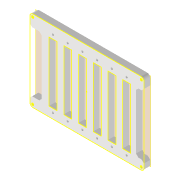
# Autodesk Inventor part: Omniscope_USBC_Base_Top+
Saved by Autodesk Inventor 2022 (Build 260153000, 153)
## iProperties
Created: 2023-05-17
Part Number: Omniscope_USBC_Base_Top+
Material: Generisch
Document SubType Name: Modeling
Designer: diederichbenedict
Density: 1 g/cm^3
Appearance: Vorgabe
Author: diederichbenedict
Autodesk Inventor part; units mm, degrees
(part 1 of 3)
ref_plane "YZ Plane" through (0, 0, 0) normal (1, 0, 0) x (0, 1, 0)
ref_plane "XZ Plane" through (0, 0, 0) normal (0, 1, 0) x (-1, 0, 0)
ref_plane "XY Plane" through (0, 0, 0) normal (0, 0, 1) x (1, 0, 0)
ref_plane "Arbeitsebene1" through (0, 0, 0) normal (0, 0, 1) x (1, 0, 0)
sketch "Skizze1" plane through (0, 0, 0) normal (0, 0, 1) x (1, 0, 0)
  line L0 (12.3616, -8.1796) -> (13.1516, -8.1796) projected
  line L1 (13.1516, -8.1796) -> (13.1516, -8.5796) projected
  line L2 (13.1516, -8.5796) -> (12.3616, -8.5796) projected
  line L3 (12.3616, -8.5796) -> (12.3616, -8.1796) projected
  line L4 (12.3616, -8.9796) -> (13.1516, -8.9796) projected
  line L5 (13.1516, -8.9796) -> (13.1516, -9.3796) projected
  line L6 (13.1516, -9.3796) -> (12.3616, -9.3796) projected
  line L7 (12.3616, -9.3796) -> (12.3616, -8.9796) projected
  line L8 (9.9166, -12.9796) -> (9.9166, -12.5796) projected
  line L9 (9.9166, -12.5796) -> (9.8216, -12.5796) projected
  line L10 (9.8216, -12.5796) -> (9.8216, -12.1796) projected
  line L11 (9.8216, -12.1796) -> (9.9166, -12.1796) projected
  line L12 (9.9166, -12.1796) -> (9.9166, -11.7796) projected
  line L13 (9.9166, -11.7796) -> (9.8216, -11.7796) projected
  line L14 (9.8216, -11.7796) -> (9.8216, -11.3796) projected
  line L15 (9.8216, -11.3796) -> (9.9166, -11.3796) projected
  line L16 (9.9166, -11.3796) -> (9.9166, -10.9796) projected
  line L17 (9.9166, -10.9796) -> (9.8216, -10.9796) projected
  line L18 (9.8216, -10.9796) -> (9.8216, -10.5796) projected
  line L19 (9.8216, -10.5796) -> (9.9166, -10.5796) projected
  line L20 (9.9166, -10.5796) -> (9.9166, -10.1796) projected
  line L21 (9.9166, -10.1796) -> (9.8216, -10.1796) projected
  line L22 (9.8216, -10.1796) -> (9.8216, -9.7796) projected
  line L23 (9.8216, -9.7796) -> (9.9166, -9.7796) projected
  line L24 (9.9166, -9.7796) -> (9.9166, -9.3796) projected
  line L25 (9.9166, -9.3796) -> (9.8216, -9.3796) projected
  line L26 (9.8216, -9.3796) -> (9.8216, -8.9796) projected
  line L27 (9.8216, -8.9796) -> (9.9166, -8.9796) projected
  line L28 (9.9166, -8.9796) -> (9.9166, -8.5796) projected
  line L29 (9.9166, -8.5796) -> (9.8216, -8.5796) projected
  line L30 (9.8216, -8.5796) -> (9.8216, -8.1796) projected
  line L31 (9.8216, -8.1796) -> (9.9166, -8.1796) projected
  line L32 (9.9166, -8.1796) -> (9.9166, -8.0296) projected
  arc A0 (10.6866, -6.9803) -> (9.9166, -8.0296) centre (11.0166, -8.0296) ccw projected
  line L33 (10.6866, -6.9803) -> (10.6866, -6.9046) projected
  line L34 (10.6866, -6.9046) -> (12.2866, -6.9046) projected
  line L35 (12.2866, -6.9046) -> (12.2866, -7.5546) projected
  line L36 (12.2866, -7.5546) -> (12.0088, -7.5546) projected
  arc A1 (12.1166, -8.0296) -> (12.0088, -7.5546) centre (11.0166, -8.0296) ccw projected
  line L37 (12.1166, -8.0296) -> (12.1166, -13.9296) projected
  arc A2 (11.6832, -14.8046) -> (12.1166, -13.9296) centre (11.0166, -13.9296) ccw projected
  line L38 (11.6832, -14.8046) -> (12.2866, -14.8046) projected
  line L39 (12.2866, -14.8046) -> (12.2866, -15.4546) projected
  line L40 (12.2866, -15.4546) -> (10.6866, -15.4546) projected
  line L41 (10.6866, -15.4546) -> (10.6866, -14.9789) projected
  arc A3 (9.9454, -14.1796) -> (10.6866, -14.9789) centre (11.0166, -13.9296) ccw projected
  line L42 (9.9454, -14.1796) -> (9.8216, -14.1796) projected
  line L43 (9.8216, -14.1796) -> (9.8216, -13.7796) projected
  line L44 (9.8216, -13.7796) -> (9.9166, -13.7796) projected
  line L45 (9.9166, -13.7796) -> (9.9166, -13.3796) projected
  line L46 (9.9166, -13.3796) -> (9.8216, -13.3796) projected
  line L47 (9.8216, -13.3796) -> (9.8216, -12.9796) projected
  line L48 (9.8216, -12.9796) -> (9.9166, -12.9796) projected
  line L49 (12.3616, -9.7796) -> (13.1516, -9.7796) projected
  line L50 (13.1516, -9.7796) -> (13.1516, -10.1796) projected
  line L51 (13.1516, -10.1796) -> (12.3616, -10.1796) projected
  line L52 (12.3616, -10.1796) -> (12.3616, -9.7796) projected
  line L53 (12.3616, -10.5796) -> (13.1516, -10.5796) projected
  line L54 (13.1516, -10.5796) -> (13.1516, -10.9796) projected
  line L55 (13.1516, -10.9796) -> (12.3616, -10.9796) projected
  line L56 (12.3616, -10.9796) -> (12.3616, -10.5796) projected
  line L57 (12.3616, -11.3796) -> (13.1516, -11.3796) projected
  line L58 (13.1516, -11.3796) -> (13.1516, -11.7796) projected
  line L59 (13.1516, -11.7796) -> (12.3616, -11.7796) projected
  line L60 (12.3616, -11.7796) -> (12.3616, -11.3796) projected
  line L61 (12.3616, -12.1796) -> (13.1516, -12.1796) projected
  line L62 (13.1516, -12.1796) -> (13.1516, -12.5796) projected
  line L63 (13.1516, -12.5796) -> (12.3616, -12.5796) projected
  line L64 (12.3616, -12.5796) -> (12.3616, -12.1796) projected
  line L65 (12.3616, -12.9796) -> (13.1516, -12.9796) projected
  line L66 (13.1516, -12.9796) -> (13.1516, -13.3796) projected
  line L67 (13.1516, -13.3796) -> (12.3616, -13.3796) projected
  line L68 (12.3616, -13.3796) -> (12.3616, -12.9796) projected
  line L69 (12.3616, -13.7796) -> (13.1516, -13.7796) projected
  line L70 (13.1516, -13.7796) -> (13.1516, -14.1796) projected
  line L71 (13.1516, -14.1796) -> (12.3616, -14.1796) projected
  line L72 (12.3616, -14.1796) -> (12.3616, -13.7796) projected
  line L73 (-47.0034, 29.7204) -> (-46.2134, 29.7204) projected
  line L74 (-46.2134, 29.7204) -> (-46.2134, 29.3204) projected
  line L75 (-46.2134, 29.3204) -> (-47.0034, 29.3204) projected
  line L76 (-47.0034, 29.3204) -> (-47.0034, 29.7204) projected
  line L77 (-47.0034, 28.9204) -> (-46.2134, 28.9204) projected
  line L78 (-46.2134, 28.9204) -> (-46.2134, 28.5204) projected
  line L79 (-46.2134, 28.5204) -> (-47.0034, 28.5204) projected
  line L80 (-47.0034, 28.5204) -> (-47.0034, 28.9204) projected
  line L81 (-47.0034, 28.1204) -> (-46.2134, 28.1204) projected
  line L82 (-46.2134, 28.1204) -> (-46.2134, 27.7204) projected
  line L83 (-46.2134, 27.7204) -> (-47.0034, 27.7204) projected
  line L84 (-47.0034, 27.7204) -> (-47.0034, 28.1204) projected
  line L85 (-47.0034, 27.3204) -> (-46.2134, 27.3204) projected
  line L86 (-46.2134, 27.3204) -> (-46.2134, 26.9204) projected
  line L87 (-46.2134, 26.9204) -> (-47.0034, 26.9204) projected
  line L88 (-47.0034, 26.9204) -> (-47.0034, 27.3204) projected
  line L89 (-47.0034, 26.5204) -> (-46.2134, 26.5204) projected
  line L90 (-46.2134, 26.5204) -> (-46.2134, 26.1204) projected
  line L91 (-46.2134, 26.1204) -> (-47.0034, 26.1204) projected
  line L92 (-47.0034, 26.1204) -> (-47.0034, 26.5204) projected
  line L93 (-47.0034, 25.7204) -> (-46.2134, 25.7204) projected
  line L94 (-46.2134, 25.7204) -> (-46.2134, 25.3204) projected
  line L95 (-46.2134, 25.3204) -> (-47.0034, 25.3204) projected
  line L96 (-47.0034, 25.3204) -> (-47.0034, 25.7204) projected
  line L97 (-47.0034, 24.9204) -> (-46.2134, 24.9204) projected
  line L98 (-46.2134, 24.9204) -> (-46.2134, 24.5204) projected
  line L99 (-46.2134, 24.5204) -> (-47.0034, 24.5204) projected
  line L100 (-47.0034, 24.5204) -> (-47.0034, 24.9204) projected
  line L101 (-47.0034, 24.1204) -> (-46.2134, 24.1204) projected
  line L102 (-46.2134, 24.1204) -> (-46.2134, 23.7204) projected
  line L103 (-46.2134, 23.7204) -> (-47.0034, 23.7204) projected
  line L104 (-47.0034, 23.7204) -> (-47.0034, 24.1204) projected
  line L105 (49.9241, -8.1296) -> (50.7141, -8.1296) projected
  line L106 (50.7141, -8.1296) -> (50.7141, -8.5296) projected
  line L107 (50.7141, -8.5296) -> (49.9241, -8.5296) projected
  line L108 (49.9241, -8.5296) -> (49.9241, -8.1296) projected
  line L109 (49.9241, -8.9296) -> (50.7141, -8.9296) projected
  line L110 (50.7141, -8.9296) -> (50.7141, -9.3296) projected
  line L111 (50.7141, -9.3296) -> (49.9241, -9.3296) projected
  line L112 (49.9241, -9.3296) -> (49.9241, -8.9296) projected
  line L113 (49.9241, -9.7296) -> (50.7141, -9.7296) projected
  line L114 (50.7141, -9.7296) -> (50.7141, -10.1296) projected
  line L115 (50.7141, -10.1296) -> (49.9241, -10.1296) projected
  line L116 (49.9241, -10.1296) -> (49.9241, -9.7296) projected
  line L117 (49.9241, -10.5296) -> (50.7141, -10.5296) projected
  line L118 (50.7141, -10.5296) -> (50.7141, -10.9296) projected
  line L119 (50.7141, -10.9296) -> (49.9241, -10.9296) projected
  line L120 (49.9241, -10.9296) -> (49.9241, -10.5296) projected
  line L121 (49.9241, -11.3296) -> (50.7141, -11.3296) projected
  line L122 (50.7141, -11.3296) -> (50.7141, -11.7296) projected
  line L123 (50.7141, -11.7296) -> (49.9241, -11.7296) projected
  line L124 (49.9241, -11.7296) -> (49.9241, -11.3296) projected
  line L125 (49.9241, -12.1296) -> (50.7141, -12.1296) projected
  line L126 (50.7141, -12.1296) -> (50.7141, -12.5296) projected
  line L127 (50.7141, -12.5296) -> (49.9241, -12.5296) projected
  line L128 (49.9241, -12.5296) -> (49.9241, -12.1296) projected
  line L129 (49.9241, -12.9296) -> (50.7141, -12.9296) projected
  line L130 (50.7141, -12.9296) -> (50.7141, -13.3296) projected
  line L131 (50.7141, -13.3296) -> (49.9241, -13.3296) projected
  line L132 (49.9241, -13.3296) -> (49.9241, -12.9296) projected
  line L133 (49.9241, -13.7296) -> (50.7141, -13.7296) projected
  line L134 (50.7141, -13.7296) -> (50.7141, -14.1296) projected
  line L135 (50.7141, -14.1296) -> (49.9241, -14.1296) projected
  line L136 (49.9241, -14.1296) -> (49.9241, -13.7296) projected
  arc A4 (49.5166, -8.0296) -> (49.3832, -7.5046) centre (48.4166, -8.0296) ccw projected
  line L137 (49.5166, -8.0296) -> (49.5166, -13.9296) projected
  arc A5 (49.1442, -14.7546) -> (49.5166, -13.9296) centre (48.4166, -13.9296) ccw projected
  line L138 (49.1442, -14.7546) -> (49.8491, -14.7546) projected
  line L139 (49.8491, -14.7546) -> (49.8491, -15.4046) projected
  line L140 (49.8491, -15.4046) -> (48.2491, -15.4046) projected
  line L141 (48.2491, -15.4046) -> (48.2491, -15.0168) projected
  arc A6 (47.3166, -13.9296) -> (48.2491, -15.0168) centre (48.4166, -13.9296) ccw projected
  line L142 (47.3166, -13.9296) -> (47.3166, -8.0296) projected
  arc A7 (48.2491, -6.9424) -> (47.3166, -8.0296) centre (48.4166, -8.0296) ccw projected
  line L143 (48.2491, -6.9424) -> (48.2491, -6.8546) projected
  line L144 (48.2491, -6.8546) -> (49.8491, -6.8546) projected
  line L145 (49.8491, -6.8546) -> (49.8491, -7.5046) projected
  line L146 (49.8491, -7.5046) -> (49.3832, -7.5046) projected
  line L147 (-46.1834, -8.0546) -> (-46.1834, -8.0296) projected
  arc A8 (-46.0054, -7.4296) -> (-46.1834, -8.0296) centre (-45.0834, -8.0296) ccw projected
  line L148 (-46.0054, -7.4296) -> (-46.0634, -7.4296) projected
  line L149 (-46.0634, -7.4296) -> (-46.0634, -6.7796) projected
  line L150 (-46.0634, -6.7796) -> (-44.4634, -6.7796) projected
  line L151 (-44.4634, -6.7796) -> (-44.4634, -7.121) projected
  arc A9 (-43.9834, -8.0296) -> (-44.4634, -7.121) centre (-45.0834, -8.0296) ccw projected
  line L152 (-43.9834, -8.0296) -> (-43.9834, -8.0546) projected
  line L153 (-43.9834, -8.0546) -> (-43.5984, -8.0546) projected
  line L154 (-43.5984, -8.0546) -> (-43.5984, -8.4546) projected
  line L155 (-43.5984, -8.4546) -> (-43.9834, -8.4546) projected
  line L156 (-43.9834, -8.4546) -> (-43.9834, -8.8546) projected
  line L157 (-43.9834, -8.8546) -> (-43.5984, -8.8546) projected
  line L158 (-43.5984, -8.8546) -> (-43.5984, -9.2546) projected
  line L159 (-43.5984, -9.2546) -> (-43.9834, -9.2546) projected
  line L160 (-43.9834, -9.2546) -> (-43.9834, -9.6546) projected
  line L161 (-43.9834, -9.6546) -> (-43.5984, -9.6546) projected
  line L162 (-43.5984, -9.6546) -> (-43.5984, -10.0546) projected
  line L163 (-43.5984, -10.0546) -> (-43.9834, -10.0546) projected
  line L164 (-43.9834, -10.0546) -> (-43.9834, -10.4546) projected
  line L165 (-43.9834, -10.4546) -> (-43.5984, -10.4546) projected
  line L166 (-43.5984, -10.4546) -> (-43.5984, -10.8546) projected
  line L167 (-43.5984, -10.8546) -> (-43.9834, -10.8546) projected
  line L168 (-43.9834, -10.8546) -> (-43.9834, -11.2546) projected
  line L169 (-43.9834, -11.2546) -> (-43.5984, -11.2546) projected
  line L170 (-43.5984, -11.2546) -> (-43.5984, -11.6546) projected
  line L171 (-43.5984, -11.6546) -> (-43.9834, -11.6546) projected
  line L172 (-43.9834, -11.6546) -> (-43.9834, -12.0546) projected
  line L173 (-43.9834, -12.0546) -> (-43.5984, -12.0546) projected
  line L174 (-43.5984, -12.0546) -> (-43.5984, -12.4546) projected
  line L175 (-43.5984, -12.4546) -> (-43.9834, -12.4546) projected
  line L176 (-43.9834, -12.4546) -> (-43.9834, -12.8546) projected
  line L177 (-43.9834, -12.8546) -> (-43.5984, -12.8546) projected
  line L178 (-43.5984, -12.8546) -> (-43.5984, -13.2546) projected
  line L179 (-43.5984, -13.2546) -> (-43.9834, -13.2546) projected
  line L180 (-43.9834, -13.2546) -> (-43.9834, -13.6546) projected
  line L181 (-43.9834, -13.6546) -> (-43.5984, -13.6546) projected
  line L182 (-43.5984, -13.6546) -> (-43.5984, -14.0546) projected
  line L183 (-43.5984, -14.0546) -> (-43.9905, -14.0546) projected
  arc A10 (-44.4634, -14.8382) -> (-43.9905, -14.0546) centre (-45.0834, -13.9296) ccw projected
  line L184 (-44.4634, -14.8382) -> (-44.4634, -15.3296) projected
  line L185 (-44.4634, -15.3296) -> (-46.0634, -15.3296) projected
  line L186 (-46.0634, -15.3296) -> (-46.0634, -14.6796) projected
  line L187 (-46.0634, -14.6796) -> (-45.8881, -14.6796) projected
  arc A11 (-46.1763, -14.0546) -> (-45.8881, -14.6796) centre (-45.0834, -13.9296) ccw projected
  line L188 (-46.1763, -14.0546) -> (-46.9284, -14.0546) projected
  line L189 (-46.9284, -14.0546) -> (-46.9284, -13.6546) projected
  line L190 (-46.9284, -13.6546) -> (-46.1834, -13.6546) projected
  line L191 (-46.1834, -13.6546) -> (-46.1834, -13.2546) projected
  line L192 (-46.1834, -13.2546) -> (-46.9284, -13.2546) projected
  line L193 (-46.9284, -13.2546) -> (-46.9284, -12.8546) projected
  line L194 (-46.9284, -12.8546) -> (-46.1834, -12.8546) projected
  line L195 (-46.1834, -12.8546) -> (-46.1834, -12.4546) projected
  line L196 (-46.1834, -12.4546) -> (-46.9284, -12.4546) projected
  line L197 (-46.9284, -12.4546) -> (-46.9284, -12.0546) projected
  line L198 (-46.9284, -12.0546) -> (-46.1834, -12.0546) projected
  line L199 (-46.1834, -12.0546) -> (-46.1834, -11.6546) projected
  line L200 (-46.1834, -11.6546) -> (-46.9284, -11.6546) projected
  line L201 (-46.9284, -11.6546) -> (-46.9284, -11.2546) projected
  line L202 (-46.9284, -11.2546) -> (-46.1834, -11.2546) projected
  line L203 (-46.1834, -11.2546) -> (-46.1834, -10.8546) projected
  line L204 (-46.1834, -10.8546) -> (-46.9284, -10.8546) projected
  line L205 (-46.9284, -10.8546) -> (-46.9284, -10.4546) projected
  line L206 (-46.9284, -10.4546) -> (-46.1834, -10.4546) projected
  line L207 (-46.1834, -10.4546) -> (-46.1834, -10.0546) projected
  line L208 (-46.1834, -10.0546) -> (-46.9284, -10.0546) projected
  line L209 (-46.9284, -10.0546) -> (-46.9284, -9.6546) projected
  line L210 (-46.9284, -9.6546) -> (-46.1834, -9.6546) projected
  line L211 (-46.1834, -9.6546) -> (-46.1834, -9.2546) projected
  line L212 (-46.1834, -9.2546) -> (-46.9284, -9.2546) projected
  line L213 (-46.9284, -9.2546) -> (-46.9284, -8.8546) projected
  line L214 (-46.9284, -8.8546) -> (-46.1834, -8.8546) projected
  line L215 (-46.1834, -8.8546) -> (-46.1834, -8.4546) projected
  line L216 (-46.1834, -8.4546) -> (-46.9284, -8.4546) projected
  line L217 (-46.9284, -8.4546) -> (-46.9284, -8.0546) projected
  line L218 (-46.9284, -8.0546) -> (-46.1834, -8.0546) projected
  line L219 (31.8441, -32.7296) -> (31.0541, -32.7296) projected
  line L220 (31.0541, -32.7296) -> (31.0541, -32.3296) projected
  line L221 (31.0541, -32.3296) -> (31.8441, -32.3296) projected
  line L222 (31.8441, -32.3296) -> (31.8441, -32.7296) projected
  line L223 (31.8441, -31.9296) -> (31.0541, -31.9296) projected
  line L224 (31.0541, -31.9296) -> (31.0541, -31.5296) projected
  line L225 (31.0541, -31.5296) -> (31.8441, -31.5296) projected
  line L226 (31.8441, -31.5296) -> (31.8441, -31.9296) projected
  line L227 (31.8441, -31.1296) -> (31.0541, -31.1296) projected
  line L228 (31.0541, -31.1296) -> (31.0541, -30.7296) projected
  line L229 (31.0541, -30.7296) -> (31.8441, -30.7296) projected
  line L230 (31.8441, -30.7296) -> (31.8441, -31.1296) projected
  line L231 (31.8441, -30.3296) -> (31.0541, -30.3296) projected
  line L232 (31.0541, -30.3296) -> (31.0541, -29.9296) projected
  line L233 (31.0541, -29.9296) -> (31.8441, -29.9296) projected
  line L234 (31.8441, -29.9296) -> (31.8441, -30.3296) projected
  line L235 (31.8441, -29.5296) -> (31.0541, -29.5296) projected
  line L236 (31.0541, -29.5296) -> (31.0541, -29.1296) projected
  line L237 (31.0541, -29.1296) -> (31.8441, -29.1296) projected
  line L238 (31.8441, -29.1296) -> (31.8441, -29.5296) projected
  line L239 (31.8441, -28.7296) -> (31.0541, -28.7296) projected
  line L240 (31.0541, -28.7296) -> (31.0541, -28.3296) projected
  line L241 (31.0541, -28.3296) -> (31.8441, -28.3296) projected
  line L242 (31.8441, -28.3296) -> (31.8441, -28.7296) projected
  line L243 (31.8441, -27.9296) -> (31.0541, -27.9296) projected
  line L244 (31.0541, -27.9296) -> (31.0541, -27.5296) projected
  line L245 (31.0541, -27.5296) -> (31.8441, -27.5296) projected
  line L246 (31.8441, -27.5296) -> (31.8441, -27.9296) projected
  line L247 (31.8441, -27.1296) -> (31.0541, -27.1296) projected
  line L248 (31.0541, -27.1296) -> (31.0541, -26.7296) projected
  line L249 (31.0541, -26.7296) -> (31.8441, -26.7296) projected
  line L250 (31.8441, -26.7296) -> (31.8441, -27.1296) projected
  line L251 (50.8941, -32.7546) -> (50.1041, -32.7546) projected
  line L252 (50.1041, -32.7546) -> (50.1041, -32.3546) projected
  line L253 (50.1041, -32.3546) -> (50.8941, -32.3546) projected
  line L254 (50.8941, -32.3546) -> (50.8941, -32.7546) projected
  line L255 (50.8941, -31.9546) -> (50.1041, -31.9546) projected
  line L256 (50.1041, -31.9546) -> (50.1041, -31.5546) projected
  line L257 (50.1041, -31.5546) -> (50.8941, -31.5546) projected
  line L258 (50.8941, -31.5546) -> (50.8941, -31.9546) projected
  line L259 (50.8941, -31.1546) -> (50.1041, -31.1546) projected
  line L260 (50.1041, -31.1546) -> (50.1041, -30.7546) projected
  line L261 (50.1041, -30.7546) -> (50.8941, -30.7546) projected
  line L262 (50.8941, -30.7546) -> (50.8941, -31.1546) projected
  line L263 (50.8941, -30.3546) -> (50.1041, -30.3546) projected
  line L264 (50.1041, -30.3546) -> (50.1041, -29.9546) projected
  line L265 (50.1041, -29.9546) -> (50.8941, -29.9546) projected
  line L266 (50.8941, -29.9546) -> (50.8941, -30.3546) projected
  line L267 (50.8941, -29.5546) -> (50.1041, -29.5546) projected
  line L268 (50.1041, -29.5546) -> (50.1041, -29.1546) projected
  line L269 (50.1041, -29.1546) -> (50.8941, -29.1546) projected
  line L270 (50.8941, -29.1546) -> (50.8941, -29.5546) projected
  line L271 (50.8941, -28.7546) -> (50.1041, -28.7546) projected
  line L272 (50.1041, -28.7546) -> (50.1041, -28.3546) projected
  line L273 (50.1041, -28.3546) -> (50.8941, -28.3546) projected
  line L274 (50.8941, -28.3546) -> (50.8941, -28.7546) projected
  line L275 (50.8941, -27.9546) -> (50.1041, -27.9546) projected
  line L276 (50.1041, -27.9546) -> (50.1041, -27.5546) projected
  line L277 (50.1041, -27.5546) -> (50.8941, -27.5546) projected
  line L278 (50.8941, -27.5546) -> (50.8941, -27.9546) projected
  line L279 (50.8941, -27.1546) -> (50.1041, -27.1546) projected
  line L280 (50.1041, -27.1546) -> (50.1041, -26.7546) projected
  line L281 (50.1041, -26.7546) -> (50.8941, -26.7546) projected
  line L282 (50.8941, -26.7546) -> (50.8941, -27.1546) projected
  arc A12 (49.5166, -26.7296) -> (49.3386, -26.1296) centre (48.4166, -26.7296) ccw projected
  line L283 (49.5166, -26.7296) -> (49.5166, -32.6296) projected
  arc A13 (49.2213, -33.3796) -> (49.5166, -32.6296) centre (48.4166, -32.6296) ccw projected
  line L284 (49.2213, -33.3796) -> (50.0291, -33.3796) projected
  line L285 (50.0291, -33.3796) -> (50.0291, -34.0296) projected
  line L286 (50.0291, -34.0296) -> (48.4291, -34.0296) projected
  line L287 (48.4291, -34.0296) -> (48.4291, -33.7295) projected
  arc A14 (47.3166, -32.6296) -> (48.4291, -33.7295) centre (48.4166, -32.6296) ccw projected
  line L288 (47.3166, -32.6296) -> (47.3166, -26.7296) projected
  arc A15 (48.4291, -25.6297) -> (47.3166, -26.7296) centre (48.4166, -26.7296) ccw projected
  line L289 (48.4291, -25.6297) -> (48.4291, -25.4796) projected
  line L290 (48.4291, -25.4796) -> (50.0291, -25.4796) projected
  line L291 (50.0291, -25.4796) -> (50.0291, -26.1296) projected
  line L292 (50.0291, -26.1296) -> (49.3386, -26.1296) projected
  line L293 (31.6866, 4.9454) -> (30.8966, 4.9454) projected
  line L294 (30.8966, 4.9454) -> (30.8966, 5.3454) projected
  line L295 (30.8966, 5.3454) -> (31.6866, 5.3454) projected
  line L296 (31.6866, 5.3454) -> (31.6866, 4.9454) projected
  line L297 (31.6866, 5.7454) -> (30.8966, 5.7454) projected
  line L298 (30.8966, 5.7454) -> (30.8966, 6.1454) projected
  line L299 (30.8966, 6.1454) -> (31.6866, 6.1454) projected
  line L300 (31.6866, 6.1454) -> (31.6866, 5.7454) projected
  line L301 (31.6866, 6.5454) -> (30.8966, 6.5454) projected
  line L302 (30.8966, 6.5454) -> (30.8966, 6.9454) projected
  line L303 (30.8966, 6.9454) -> (31.6866, 6.9454) projected
  line L304 (31.6866, 6.9454) -> (31.6866, 6.5454) projected
  line L305 (31.6866, 7.3454) -> (30.8966, 7.3454) projected
  line L306 (30.8966, 7.3454) -> (30.8966, 7.7454) projected
  line L307 (30.8966, 7.7454) -> (31.6866, 7.7454) projected
  line L308 (31.6866, 7.7454) -> (31.6866, 7.3454) projected
  line L309 (31.6866, 8.1454) -> (30.8966, 8.1454) projected
  line L310 (30.8966, 8.1454) -> (30.8966, 8.5454) projected
  line L311 (30.8966, 8.5454) -> (31.6866, 8.5454) projected
  line L312 (31.6866, 8.5454) -> (31.6866, 8.1454) projected
  line L313 (31.6866, 8.9454) -> (30.8966, 8.9454) projected
  line L314 (30.8966, 8.9454) -> (30.8966, 9.3454) projected
  line L315 (30.8966, 9.3454) -> (31.6866, 9.3454) projected
  line L316 (31.6866, 9.3454) -> (31.6866, 8.9454) projected
  line L317 (31.6866, 9.7454) -> (30.8966, 9.7454) projected
  line L318 (30.8966, 9.7454) -> (30.8966, 10.1454) projected
  line L319 (30.8966, 10.1454) -> (31.6866, 10.1454) projected
  line L320 (31.6866, 10.1454) -> (31.6866, 9.7454) projected
  line L321 (31.6866, 10.5454) -> (30.8966, 10.5454) projected
  line L322 (30.8966, 10.5454) -> (30.8966, 10.9454) projected
  line L323 (30.8966, 10.9454) -> (31.6866, 10.9454) projected
  line L324 (31.6866, 10.9454) -> (31.6866, 10.5454) projected
  line L325 (13.0191, -32.6296) -> (12.2291, -32.6296) projected
  line L326 (12.2291, -32.6296) -> (12.2291, -32.2296) projected
  line L327 (12.2291, -32.2296) -> (13.0191, -32.2296) projected
  line L328 (13.0191, -32.2296) -> (13.0191, -32.6296) projected
  line L329 (13.0191, -31.8296) -> (12.2291, -31.8296) projected
  line L330 (12.2291, -31.8296) -> (12.2291, -31.4296) projected
  line L331 (12.2291, -31.4296) -> (13.0191, -31.4296) projected
  line L332 (13.0191, -31.4296) -> (13.0191, -31.8296) projected
  line L333 (13.0191, -31.0296) -> (12.2291, -31.0296) projected
  line L334 (12.2291, -31.0296) -> (12.2291, -30.6296) projected
  line L335 (12.2291, -30.6296) -> (13.0191, -30.6296) projected
  line L336 (13.0191, -30.6296) -> (13.0191, -31.0296) projected
  line L337 (13.0191, -30.2296) -> (12.2291, -30.2296) projected
  line L338 (12.2291, -30.2296) -> (12.2291, -29.8296) projected
  line L339 (12.2291, -29.8296) -> (13.0191, -29.8296) projected
  line L340 (13.0191, -29.8296) -> (13.0191, -30.2296) projected
  line L341 (13.0191, -29.4296) -> (12.2291, -29.4296) projected
  line L342 (12.2291, -29.4296) -> (12.2291, -29.0296) projected
  line L343 (12.2291, -29.0296) -> (13.0191, -29.0296) projected
  line L344 (13.0191, -29.0296) -> (13.0191, -29.4296) projected
  line L345 (13.0191, -28.6296) -> (12.2291, -28.6296) projected
  line L346 (12.2291, -28.6296) -> (12.2291, -28.2296) projected
  line L347 (12.2291, -28.2296) -> (13.0191, -28.2296) projected
  line L348 (13.0191, -28.2296) -> (13.0191, -28.6296) projected
  line L349 (13.0191, -27.8296) -> (12.2291, -27.8296) projected
  line L350 (12.2291, -27.8296) -> (12.2291, -27.4296) projected
  line L351 (12.2291, -27.4296) -> (13.0191, -27.4296) projected
  line L352 (13.0191, -27.4296) -> (13.0191, -27.8296) projected
  line L353 (13.0191, -27.0296) -> (12.2291, -27.0296) projected
  line L354 (12.2291, -27.0296) -> (12.2291, -26.6296) projected
  line L355 (12.2291, -26.6296) -> (13.0191, -26.6296) projected
  line L356 (13.0191, -26.6296) -> (13.0191, -27.0296) projected
  line L357 (-27.4834, -8.0796) -> (-27.4834, -8.0296) projected
  arc A16 (-27.0134, -7.1279) -> (-27.4834, -8.0296) centre (-26.3834, -8.0296) ccw projected
  line L358 (-27.0134, -7.1279) -> (-27.0134, -6.8046) projected
  line L359 (-27.0134, -6.8046) -> (-25.4134, -6.8046) projected
  line L360 (-25.4134, -6.8046) -> (-25.4134, -7.4546) projected
  line L361 (-25.4134, -7.4546) -> (-25.4457, -7.4546) projected
  arc A17 (-25.2834, -8.0296) -> (-25.4457, -7.4546) centre (-26.3834, -8.0296) ccw projected
  line L362 (-25.2834, -8.0296) -> (-25.2834, -8.0796) projected
  line L363 (-25.2834, -8.0796) -> (-24.5484, -8.0796) projected
  line L364 (-24.5484, -8.0796) -> (-24.5484, -8.4796) projected
  line L365 (-24.5484, -8.4796) -> (-25.2834, -8.4796) projected
  line L366 (-25.2834, -8.4796) -> (-25.2834, -8.8796) projected
  line L367 (-25.2834, -8.8796) -> (-24.5484, -8.8796) projected
  line L368 (-24.5484, -8.8796) -> (-24.5484, -9.2796) projected
  line L369 (-24.5484, -9.2796) -> (-25.2834, -9.2796) projected
  line L370 (-25.2834, -9.2796) -> (-25.2834, -9.6796) projected
  line L371 (-25.2834, -9.6796) -> (-24.5484, -9.6796) projected
  line L372 (-24.5484, -9.6796) -> (-24.5484, -10.0796) projected
  line L373 (-24.5484, -10.0796) -> (-25.2834, -10.0796) projected
  line L374 (-25.2834, -10.0796) -> (-25.2834, -10.4796) projected
  line L375 (-25.2834, -10.4796) -> (-24.5484, -10.4796) projected
  line L376 (-24.5484, -10.4796) -> (-24.5484, -10.8796) projected
  line L377 (-24.5484, -10.8796) -> (-25.2834, -10.8796) projected
  line L378 (-25.2834, -10.8796) -> (-25.2834, -11.2796) projected
  line L379 (-25.2834, -11.2796) -> (-24.5484, -11.2796) projected
  line L380 (-24.5484, -11.2796) -> (-24.5484, -11.6796) projected
  line L381 (-24.5484, -11.6796) -> (-25.2834, -11.6796) projected
  line L382 (-25.2834, -11.6796) -> (-25.2834, -12.0796) projected
  line L383 (-25.2834, -12.0796) -> (-24.5484, -12.0796) projected
  line L384 (-24.5484, -12.0796) -> (-24.5484, -12.4796) projected
  line L385 (-24.5484, -12.4796) -> (-25.2834, -12.4796) projected
  line L386 (-25.2834, -12.4796) -> (-25.2834, -12.8796) projected
  line L387 (-25.2834, -12.8796) -> (-24.5484, -12.8796) projected
  line L388 (-24.5484, -12.8796) -> (-24.5484, -13.2796) projected
  line L389 (-24.5484, -13.2796) -> (-25.2834, -13.2796) projected
  line L390 (-25.2834, -13.2796) -> (-25.2834, -13.6796) projected
  line L391 (-25.2834, -13.6796) -> (-24.5484, -13.6796) projected
  line L392 (-24.5484, -13.6796) -> (-24.5484, -14.0796) projected
  line L393 (-24.5484, -14.0796) -> (-25.2937, -14.0796) projected
  arc A18 (-25.6028, -14.7046) -> (-25.2937, -14.0796) centre (-26.3834, -13.9296) ccw projected
  line L394 (-25.6028, -14.7046) -> (-25.4134, -14.7046) projected
  line L395 (-25.4134, -14.7046) -> (-25.4134, -15.3546) projected
  line L396 (-25.4134, -15.3546) -> (-27.0134, -15.3546) projected
  line L397 (-27.0134, -15.3546) -> (-27.0134, -14.8313) projected
  arc A19 (-27.4731, -14.0796) -> (-27.0134, -14.8313) centre (-26.3834, -13.9296) ccw projected
  line L398 (-27.4731, -14.0796) -> (-27.8784, -14.0796) projected
  line L399 (-27.8784, -14.0796) -> (-27.8784, -13.6796) projected
  line L400 (-27.8784, -13.6796) -> (-27.4834, -13.6796) projected
  line L401 (-27.4834, -13.6796) -> (-27.4834, -13.2796) projected
  line L402 (-27.4834, -13.2796) -> (-27.8784, -13.2796) projected
  line L403 (-27.8784, -13.2796) -> (-27.8784, -12.8796) projected
  line L404 (-27.8784, -12.8796) -> (-27.4834, -12.8796) projected
  line L405 (-27.4834, -12.8796) -> (-27.4834, -12.4796) projected
  line L406 (-27.4834, -12.4796) -> (-27.8784, -12.4796) projected
  line L407 (-27.8784, -12.4796) -> (-27.8784, -12.0796) projected
  line L408 (-27.8784, -12.0796) -> (-27.4834, -12.0796) projected
  line L409 (-27.4834, -12.0796) -> (-27.4834, -11.6796) projected
  line L410 (-27.4834, -11.6796) -> (-27.8784, -11.6796) projected
  line L411 (-27.8784, -11.6796) -> (-27.8784, -11.2796) projected
  line L412 (-27.8784, -11.2796) -> (-27.4834, -11.2796) projected
  line L413 (-27.4834, -11.2796) -> (-27.4834, -10.8796) projected
  line L414 (-27.4834, -10.8796) -> (-27.8784, -10.8796) projected
  line L415 (-27.8784, -10.8796) -> (-27.8784, -10.4796) projected
  line L416 (-27.8784, -10.4796) -> (-27.4834, -10.4796) projected
  line L417 (-27.4834, -10.4796) -> (-27.4834, -10.0796) projected
  line L418 (-27.4834, -10.0796) -> (-27.8784, -10.0796) projected
  line L419 (-27.8784, -10.0796) -> (-27.8784, -9.6796) projected
  line L420 (-27.8784, -9.6796) -> (-27.4834, -9.6796) projected
  line L421 (-27.4834, -9.6796) -> (-27.4834, -9.2796) projected
  line L422 (-27.4834, -9.2796) -> (-27.8784, -9.2796) projected
  line L423 (-27.8784, -9.2796) -> (-27.8784, -8.8796) projected
  line L424 (-27.8784, -8.8796) -> (-27.4834, -8.8796) projected
  line L425 (-27.4834, -8.8796) -> (-27.4834, -8.4796) projected
  line L426 (-27.4834, -8.4796) -> (-27.8784, -8.4796) projected
  line L427 (-27.8784, -8.4796) -> (-27.8784, -8.0796) projected
  line L428 (-27.8784, -8.0796) -> (-27.4834, -8.0796) projected
  line L429 (49.8491, 29.6454) -> (50.6391, 29.6454) projected
  line L430 (50.6391, 29.6454) -> (50.6391, 29.2454) projected
  line L431 (50.6391, 29.2454) -> (49.8491, 29.2454) projected
  line L432 (49.8491, 29.2454) -> (49.8491, 29.6454) projected
  line L433 (49.8491, 28.8454) -> (50.6391, 28.8454) projected
  line L434 (50.6391, 28.8454) -> (50.6391, 28.4454) projected
  line L435 (50.6391, 28.4454) -> (49.8491, 28.4454) projected
  line L436 (49.8491, 28.4454) -> (49.8491, 28.8454) projected
  line L437 (49.8491, 28.0454) -> (50.6391, 28.0454) projected
  line L438 (50.6391, 28.0454) -> (50.6391, 27.6454) projected
  line L439 (50.6391, 27.6454) -> (49.8491, 27.6454) projected
  line L440 (49.8491, 27.6454) -> (49.8491, 28.0454) projected
  line L441 (49.8491, 27.2454) -> (50.6391, 27.2454) projected
  line L442 (50.6391, 27.2454) -> (50.6391, 26.8454) projected
  line L443 (50.6391, 26.8454) -> (49.8491, 26.8454) projected
  line L444 (49.8491, 26.8454) -> (49.8491, 27.2454) projected
  line L445 (49.8491, 26.4454) -> (50.6391, 26.4454) projected
  line L446 (50.6391, 26.4454) -> (50.6391, 26.0454) projected
  line L447 (50.6391, 26.0454) -> (49.8491, 26.0454) projected
  line L448 (49.8491, 26.0454) -> (49.8491, 26.4454) projected
  line L449 (49.8491, 25.6454) -> (50.6391, 25.6454) projected
  line L450 (50.6391, 25.6454) -> (50.6391, 25.2454) projected
  line L451 (50.6391, 25.2454) -> (49.8491, 25.2454) projected
  line L452 (49.8491, 25.2454) -> (49.8491, 25.6454) projected
  line L453 (49.8491, 24.8454) -> (50.6391, 24.8454) projected
  line L454 (50.6391, 24.8454) -> (50.6391, 24.4454) projected
  line L455 (50.6391, 24.4454) -> (49.8491, 24.4454) projected
  line L456 (49.8491, 24.4454) -> (49.8491, 24.8454) projected
  line L457 (49.8491, 24.0454) -> (50.6391, 24.0454) projected
  line L458 (50.6391, 24.0454) -> (50.6391, 23.6454) projected
  line L459 (50.6391, 23.6454) -> (49.8491, 23.6454) projected
  line L460 (49.8491, 23.6454) -> (49.8491, 24.0454) projected
  line L461 (31.0941, 29.6704) -> (31.8841, 29.6704) projected
  line L462 (31.8841, 29.6704) -> (31.8841, 29.2704) projected
  line L463 (31.8841, 29.2704) -> (31.0941, 29.2704) projected
  line L464 (31.0941, 29.2704) -> (31.0941, 29.6704) projected
  line L465 (31.0941, 28.8704) -> (31.8841, 28.8704) projected
  line L466 (31.8841, 28.8704) -> (31.8841, 28.4704) projected
  line L467 (31.8841, 28.4704) -> (31.0941, 28.4704) projected
  line L468 (31.0941, 28.4704) -> (31.0941, 28.8704) projected
  line L469 (31.0941, 28.0704) -> (31.8841, 28.0704) projected
  line L470 (31.8841, 28.0704) -> (31.8841, 27.6704) projected
  line L471 (31.8841, 27.6704) -> (31.0941, 27.6704) projected
  line L472 (31.0941, 27.6704) -> (31.0941, 28.0704) projected
  line L473 (31.0941, 27.2704) -> (31.8841, 27.2704) projected
  line L474 (31.8841, 27.2704) -> (31.8841, 26.8704) projected
  line L475 (31.8841, 26.8704) -> (31.0941, 26.8704) projected
  line L476 (31.0941, 26.8704) -> (31.0941, 27.2704) projected
  line L477 (31.0941, 26.4704) -> (31.8841, 26.4704) projected
  line L478 (31.8841, 26.4704) -> (31.8841, 26.0704) projected
  line L479 (31.8841, 26.0704) -> (31.0941, 26.0704) projected
  line L480 (31.0941, 26.0704) -> (31.0941, 26.4704) projected
  line L481 (31.0941, 25.6704) -> (31.8841, 25.6704) projected
  line L482 (31.8841, 25.6704) -> (31.8841, 25.2704) projected
  line L483 (31.8841, 25.2704) -> (31.0941, 25.2704) projected
  line L484 (31.0941, 25.2704) -> (31.0941, 25.6704) projected
  line L485 (31.0941, 24.8704) -> (31.8841, 24.8704) projected
  line L486 (31.8841, 24.8704) -> (31.8841, 24.4704) projected
  line L487 (31.8841, 24.4704) -> (31.0941, 24.4704) projected
  line L488 (31.0941, 24.4704) -> (31.0941, 24.8704) projected
  line L489 (31.0941, 24.0704) -> (31.8841, 24.0704) projected
  line L490 (31.8841, 24.0704) -> (31.8841, 23.6704) projected
  line L491 (31.8841, 23.6704) -> (31.0941, 23.6704) projected
  line L492 (31.0941, 23.6704) -> (31.0941, 24.0704) projected
  line L493 (50.7366, 4.9204) -> (49.9466, 4.9204) projected
  line L494 (49.9466, 4.9204) -> (49.9466, 5.3204) projected
  line L495 (49.9466, 5.3204) -> (50.7366, 5.3204) projected
  line L496 (50.7366, 5.3204) -> (50.7366, 4.9204) projected
  line L497 (50.7366, 5.7204) -> (49.9466, 5.7204) projected
  line L498 (49.9466, 5.7204) -> (49.9466, 6.1204) projected
  line L499 (49.9466, 6.1204) -> (50.7366, 6.1204) projected
  line L500 (50.7366, 6.1204) -> (50.7366, 5.7204) projected
  line L501 (50.7366, 6.5204) -> (49.9466, 6.5204) projected
  line L502 (49.9466, 6.5204) -> (49.9466, 6.9204) projected
  line L503 (49.9466, 6.9204) -> (50.7366, 6.9204) projected
  line L504 (50.7366, 6.9204) -> (50.7366, 6.5204) projected
  line L505 (50.7366, 7.3204) -> (49.9466, 7.3204) projected
  line L506 (49.9466, 7.3204) -> (49.9466, 7.7204) projected
  line L507 (49.9466, 7.7204) -> (50.7366, 7.7204) projected
  line L508 (50.7366, 7.7204) -> (50.7366, 7.3204) projected
  line L509 (50.7366, 8.1204) -> (49.9466, 8.1204) projected
  line L510 (49.9466, 8.1204) -> (49.9466, 8.5204) projected
  line L511 (49.9466, 8.5204) -> (50.7366, 8.5204) projected
  line L512 (50.7366, 8.5204) -> (50.7366, 8.1204) projected
  line L513 (50.7366, 8.9204) -> (49.9466, 8.9204) projected
  line L514 (49.9466, 8.9204) -> (49.9466, 9.3204) projected
  line L515 (49.9466, 9.3204) -> (50.7366, 9.3204) projected
  line L516 (50.7366, 9.3204) -> (50.7366, 8.9204) projected
  line L517 (50.7366, 9.7204) -> (49.9466, 9.7204) projected
  line L518 (49.9466, 9.7204) -> (49.9466, 10.1204) projected
  line L519 (49.9466, 10.1204) -> (50.7366, 10.1204) projected
  line L520 (50.7366, 10.1204) -> (50.7366, 9.7204) projected
  line L521 (50.7366, 10.5204) -> (49.9466, 10.5204) projected
  line L522 (49.9466, 10.5204) -> (49.9466, 10.9204) projected
  line L523 (49.9466, 10.9204) -> (50.7366, 10.9204) projected
  line L524 (50.7366, 10.9204) -> (50.7366, 10.5204) projected
  arc A20 (49.5166, 10.6704) -> (49.0832, 11.5454) centre (48.4166, 10.6704) ccw projected
  line L525 (49.5166, 10.6704) -> (49.5166, 4.7704) projected
  arc A21 (49.4088, 4.2954) -> (49.5166, 4.7704) centre (48.4166, 4.7704) ccw projected
  line L526 (49.4088, 4.2954) -> (49.8716, 4.2954) projected
  line L527 (49.8716, 4.2954) -> (49.8716, 3.6454) projected
  line L528 (49.8716, 3.6454) -> (48.2716, 3.6454) projected
  line L529 (48.2716, 3.6454) -> (48.2716, 3.68) projected
  arc A22 (47.3166, 4.7704) -> (48.2716, 3.68) centre (48.4166, 4.7704) ccw projected
  line L530 (47.3166, 4.7704) -> (47.3166, 10.6704) projected
  arc A23 (48.2716, 11.7608) -> (47.3166, 10.6704) centre (48.4166, 10.6704) ccw projected
  line L531 (48.2716, 11.7608) -> (48.2716, 12.1954) projected
  line L532 (48.2716, 12.1954) -> (49.8716, 12.1954) projected
  line L533 (49.8716, 12.1954) -> (49.8716, 11.5454) projected
  line L534 (49.8716, 11.5454) -> (49.0832, 11.5454) projected
  line L535 (-6.5134, -8.1796) -> (-5.7234, -8.1796) projected
  line L536 (-5.7234, -8.1796) -> (-5.7234, -8.5796) projected
  line L537 (-5.7234, -8.5796) -> (-6.5134, -8.5796) projected
  line L538 (-6.5134, -8.5796) -> (-6.5134, -8.1796) projected
  line L539 (-6.5134, -8.9796) -> (-5.7234, -8.9796) projected
  line L540 (-5.7234, -8.9796) -> (-5.7234, -9.3796) projected
  line L541 (-5.7234, -9.3796) -> (-6.5134, -9.3796) projected
  line L542 (-6.5134, -9.3796) -> (-6.5134, -8.9796) projected
  line L543 (-8.7834, -12.9796) -> (-8.7834, -12.5796) projected
  line L544 (-8.7834, -12.5796) -> (-9.0534, -12.5796) projected
  line L545 (-9.0534, -12.5796) -> (-9.0534, -12.1796) projected
  line L546 (-9.0534, -12.1796) -> (-8.7834, -12.1796) projected
  line L547 (-8.7834, -12.1796) -> (-8.7834, -11.7796) projected
  line L548 (-8.7834, -11.7796) -> (-9.0534, -11.7796) projected
  line L549 (-9.0534, -11.7796) -> (-9.0534, -11.3796) projected
  line L550 (-9.0534, -11.3796) -> (-8.7834, -11.3796) projected
  line L551 (-8.7834, -11.3796) -> (-8.7834, -10.9796) projected
  line L552 (-8.7834, -10.9796) -> (-9.0534, -10.9796) projected
  line L553 (-9.0534, -10.9796) -> (-9.0534, -10.5796) projected
  line L554 (-9.0534, -10.5796) -> (-8.7834, -10.5796) projected
  line L555 (-8.7834, -10.5796) -> (-8.7834, -10.1796) projected
  line L556 (-8.7834, -10.1796) -> (-9.0534, -10.1796) projected
  line L557 (-9.0534, -10.1796) -> (-9.0534, -9.7796) projected
  line L558 (-9.0534, -9.7796) -> (-8.7834, -9.7796) projected
  line L559 (-8.7834, -9.7796) -> (-8.7834, -9.3796) projected
  line L560 (-8.7834, -9.3796) -> (-9.0534, -9.3796) projected
  line L561 (-9.0534, -9.3796) -> (-9.0534, -8.9796) projected
  line L562 (-9.0534, -8.9796) -> (-8.7834, -8.9796) projected
  line L563 (-8.7834, -8.9796) -> (-8.7834, -8.5796) projected
  line L564 (-8.7834, -8.5796) -> (-9.0534, -8.5796) projected
  line L565 (-9.0534, -8.5796) -> (-9.0534, -8.1796) projected
  line L566 (-9.0534, -8.1796) -> (-8.7834, -8.1796) projected
  line L567 (-8.7834, -8.1796) -> (-8.7834, -8.0296) projected
  arc A24 (-8.1884, -7.0524) -> (-8.7834, -8.0296) centre (-7.6834, -8.0296) ccw projected
  line L568 (-8.1884, -7.0524) -> (-8.1884, -6.9046) projected
  line L569 (-8.1884, -6.9046) -> (-6.5884, -6.9046) projected
  line L570 (-6.5884, -6.9046) -> (-6.5884, -7.5546) projected
  line L571 (-6.5884, -7.5546) -> (-6.6912, -7.5546) projected
  arc A25 (-6.5834, -8.0296) -> (-6.6912, -7.5546) centre (-7.6834, -8.0296) ccw projected
  line L572 (-6.5834, -8.0296) -> (-6.5834, -13.9296) projected
  arc A26 (-7.0168, -14.8046) -> (-6.5834, -13.9296) centre (-7.6834, -13.9296) ccw projected
  line L573 (-7.0168, -14.8046) -> (-6.5884, -14.8046) projected
  line L574 (-6.5884, -14.8046) -> (-6.5884, -15.4546) projected
  line L575 (-6.5884, -15.4546) -> (-8.1884, -15.4546) projected
  line L576 (-8.1884, -15.4546) -> (-8.1884, -14.9068) projected
  arc A27 (-8.7546, -14.1796) -> (-8.1884, -14.9068) centre (-7.6834, -13.9296) ccw projected
  line L577 (-8.7546, -14.1796) -> (-9.0534, -14.1796) projected
  line L578 (-9.0534, -14.1796) -> (-9.0534, -13.7796) projected
  line L579 (-9.0534, -13.7796) -> (-8.7834, -13.7796) projected
  line L580 (-8.7834, -13.7796) -> (-8.7834, -13.3796) projected
  line L581 (-8.7834, -13.3796) -> (-9.0534, -13.3796) projected
  line L582 (-9.0534, -13.3796) -> (-9.0534, -12.9796) projected
  line L583 (-9.0534, -12.9796) -> (-8.7834, -12.9796) projected
  line L584 (-6.5134, -9.7796) -> (-5.7234, -9.7796) projected
  line L585 (-5.7234, -9.7796) -> (-5.7234, -10.1796) projected
  line L586 (-5.7234, -10.1796) -> (-6.5134, -10.1796) projected
  line L587 (-6.5134, -10.1796) -> (-6.5134, -9.7796) projected
  line L588 (-6.5134, -10.5796) -> (-5.7234, -10.5796) projected
  line L589 (-5.7234, -10.5796) -> (-5.7234, -10.9796) projected
  line L590 (-5.7234, -10.9796) -> (-6.5134, -10.9796) projected
  line L591 (-6.5134, -10.9796) -> (-6.5134, -10.5796) projected
  line L592 (-6.5134, -11.3796) -> (-5.7234, -11.3796) projected
  line L593 (-5.7234, -11.3796) -> (-5.7234, -11.7796) projected
  line L594 (-5.7234, -11.7796) -> (-6.5134, -11.7796) projected
  line L595 (-6.5134, -11.7796) -> (-6.5134, -11.3796) projected
  line L596 (-6.5134, -12.1796) -> (-5.7234, -12.1796) projected
  line L597 (-5.7234, -12.1796) -> (-5.7234, -12.5796) projected
  line L598 (-5.7234, -12.5796) -> (-6.5134, -12.5796) projected
  line L599 (-6.5134, -12.5796) -> (-6.5134, -12.1796) projected
  line L600 (-6.5134, -12.9796) -> (-5.7234, -12.9796) projected
  line L601 (-5.7234, -12.9796) -> (-5.7234, -13.3796) projected
  line L602 (-5.7234, -13.3796) -> (-6.5134, -13.3796) projected
  line L603 (-6.5134, -13.3796) -> (-6.5134, -12.9796) projected
  line L604 (-6.5134, -13.7796) -> (-5.7234, -13.7796) projected
  line L605 (-5.7234, -13.7796) -> (-5.7234, -14.1796) projected
  line L606 (-5.7234, -14.1796) -> (-6.5134, -14.1796) projected
  line L607 (-6.5134, -14.1796) -> (-6.5134, -13.7796) projected
  line L608 (12.2866, 29.5954) -> (13.0766, 29.5954) projected
  line L609 (13.0766, 29.5954) -> (13.0766, 29.1954) projected
  line L610 (13.0766, 29.1954) -> (12.2866, 29.1954) projected
  line L611 (12.2866, 29.1954) -> (12.2866, 29.5954) projected
  line L612 (12.2866, 28.7954) -> (13.0766, 28.7954) projected
  line L613 (13.0766, 28.7954) -> (13.0766, 28.3954) projected
  line L614 (13.0766, 28.3954) -> (12.2866, 28.3954) projected
  line L615 (12.2866, 28.3954) -> (12.2866, 28.7954) projected
  line L616 (12.2866, 27.9954) -> (13.0766, 27.9954) projected
  line L617 (13.0766, 27.9954) -> (13.0766, 27.5954) projected
  line L618 (13.0766, 27.5954) -> (12.2866, 27.5954) projected
  line L619 (12.2866, 27.5954) -> (12.2866, 27.9954) projected
  line L620 (12.2866, 27.1954) -> (13.0766, 27.1954) projected
  line L621 (13.0766, 27.1954) -> (13.0766, 26.7954) projected
  line L622 (13.0766, 26.7954) -> (12.2866, 26.7954) projected
  line L623 (12.2866, 26.7954) -> (12.2866, 27.1954) projected
  line L624 (12.2866, 26.3954) -> (13.0766, 26.3954) projected
  line L625 (13.0766, 26.3954) -> (13.0766, 25.9954) projected
  line L626 (13.0766, 25.9954) -> (12.2866, 25.9954) projected
  line L627 (12.2866, 25.9954) -> (12.2866, 26.3954) projected
  line L628 (12.2866, 25.5954) -> (13.0766, 25.5954) projected
  line L629 (13.0766, 25.5954) -> (13.0766, 25.1954) projected
  line L630 (13.0766, 25.1954) -> (12.2866, 25.1954) projected
  line L631 (12.2866, 25.1954) -> (12.2866, 25.5954) projected
  line L632 (12.2866, 24.7954) -> (13.0766, 24.7954) projected
  line L633 (13.0766, 24.7954) -> (13.0766, 24.3954) projected
  line L634 (13.0766, 24.3954) -> (12.2866, 24.3954) projected
  line L635 (12.2866, 24.3954) -> (12.2866, 24.7954) projected
  line L636 (12.2866, 23.9954) -> (13.0766, 23.9954) projected
  line L637 (13.0766, 23.9954) -> (13.0766, 23.5954) projected
  line L638 (13.0766, 23.5954) -> (12.2866, 23.5954) projected
  line L639 (12.2866, 23.5954) -> (12.2866, 23.9954) projected
  line L640 (31.1691, -8.1046) -> (31.9591, -8.1046) projected
  line L641 (31.9591, -8.1046) -> (31.9591, -8.5046) projected
  line L642 (31.9591, -8.5046) -> (31.1691, -8.5046) projected
  line L643 (31.1691, -8.5046) -> (31.1691, -8.1046) projected
  line L644 (31.1691, -8.9046) -> (31.9591, -8.9046) projected
  line L645 (31.9591, -8.9046) -> (31.9591, -9.3046) projected
  line L646 (31.9591, -9.3046) -> (31.1691, -9.3046) projected
  line L647 (31.1691, -9.3046) -> (31.1691, -8.9046) projected
  line L648 (31.1691, -9.7046) -> (31.9591, -9.7046) projected
  line L649 (31.9591, -9.7046) -> (31.9591, -10.1046) projected
  line L650 (31.9591, -10.1046) -> (31.1691, -10.1046) projected
  line L651 (31.1691, -10.1046) -> (31.1691, -9.7046) projected
  line L652 (31.1691, -10.5046) -> (31.9591, -10.5046) projected
  line L653 (31.9591, -10.5046) -> (31.9591, -10.9046) projected
  line L654 (31.9591, -10.9046) -> (31.1691, -10.9046) projected
  line L655 (31.1691, -10.9046) -> (31.1691, -10.5046) projected
  line L656 (31.1691, -11.3046) -> (31.9591, -11.3046) projected
  line L657 (31.9591, -11.3046) -> (31.9591, -11.7046) projected
  line L658 (31.9591, -11.7046) -> (31.1691, -11.7046) projected
  line L659 (31.1691, -11.7046) -> (31.1691, -11.3046) projected
  line L660 (31.1691, -12.1046) -> (31.9591, -12.1046) projected
  line L661 (31.9591, -12.1046) -> (31.9591, -12.5046) projected
  line L662 (31.9591, -12.5046) -> (31.1691, -12.5046) projected
  line L663 (31.1691, -12.5046) -> (31.1691, -12.1046) projected
  line L664 (31.1691, -12.9046) -> (31.9591, -12.9046) projected
  line L665 (31.9591, -12.9046) -> (31.9591, -13.3046) projected
  line L666 (31.9591, -13.3046) -> (31.1691, -13.3046) projected
  line L667 (31.1691, -13.3046) -> (31.1691, -12.9046) projected
  line L668 (31.1691, -13.7046) -> (31.9591, -13.7046) projected
  line L669 (31.9591, -13.7046) -> (31.9591, -14.1046) projected
  line L670 (31.9591, -14.1046) -> (31.1691, -14.1046) projected
  line L671 (31.1691, -14.1046) -> (31.1691, -13.7046) projected
  line L672 (66.421, 45.4152) -> (-66.421, 45.4152) projected
  line L673 (-66.421, 45.4152) -> (-66.421, -45.4152) projected
  line L674 (-66.421, -45.4152) -> (66.421, -45.4152) projected
  line L675 (66.421, -45.4152) -> (66.421, 45.4152) projected
  line L676 (-43.9834, -31.8796) -> (-43.9834, -32.2796) projected
  line L677 (-43.9834, -32.2796) -> (-43.4184, -32.2796) projected
  line L678 (-43.4184, -32.2796) -> (-43.4184, -32.6796) projected
  line L679 (-43.4184, -32.6796) -> (-43.9845, -32.6796) projected
  arc A28 (-44.2834, -33.3846) -> (-43.9845, -32.6796) centre (-45.0834, -32.6296) ccw projected
  line L680 (-44.2834, -33.3846) -> (-44.2834, -33.9546) projected
  line L681 (-44.2834, -33.9546) -> (-45.8834, -33.9546) projected
  line L682 (-45.8834, -33.9546) -> (-45.8834, -33.3846) projected
  arc A29 (-46.1823, -32.6796) -> (-45.8834, -33.3846) centre (-45.0834, -32.6296) ccw projected
  line L683 (-46.1823, -32.6796) -> (-46.7484, -32.6796) projected
  line L684 (-46.7484, -32.6796) -> (-46.7484, -32.2796) projected
  line L685 (-46.7484, -32.2796) -> (-46.1834, -32.2796) projected
  line L686 (-46.1834, -32.2796) -> (-46.1834, -31.8796) projected
  line L687 (-46.1834, -31.8796) -> (-46.7484, -31.8796) projected
  line L688 (-46.7484, -31.8796) -> (-46.7484, -31.4796) projected
  line L689 (-46.7484, -31.4796) -> (-46.1834, -31.4796) projected
  line L690 (-46.1834, -31.4796) -> (-46.1834, -31.0796) projected
  line L691 (-46.1834, -31.0796) -> (-46.7484, -31.0796) projected
  line L692 (-46.7484, -31.0796) -> (-46.7484, -30.6796) projected
  line L693 (-46.7484, -30.6796) -> (-46.1834, -30.6796) projected
  line L694 (-46.1834, -30.6796) -> (-46.1834, -30.2796) projected
  line L695 (-46.1834, -30.2796) -> (-46.7484, -30.2796) projected
  line L696 (-46.7484, -30.2796) -> (-46.7484, -29.8796) projected
  line L697 (-46.7484, -29.8796) -> (-46.1834, -29.8796) projected
  line L698 (-46.1834, -29.8796) -> (-46.1834, -29.4796) projected
  line L699 (-46.1834, -29.4796) -> (-46.7484, -29.4796) projected
  line L700 (-46.7484, -29.4796) -> (-46.7484, -29.0796) projected
  line L701 (-46.7484, -29.0796) -> (-46.1834, -29.0796) projected
  line L702 (-46.1834, -29.0796) -> (-46.1834, -28.6796) projected
  line L703 (-46.1834, -28.6796) -> (-46.7484, -28.6796) projected
  line L704 (-46.7484, -28.6796) -> (-46.7484, -28.2796) projected
  line L705 (-46.7484, -28.2796) -> (-46.1834, -28.2796) projected
  line L706 (-46.1834, -28.2796) -> (-46.1834, -27.8796) projected
  line L707 (-46.1834, -27.8796) -> (-46.7484, -27.8796) projected
  line L708 (-46.7484, -27.8796) -> (-46.7484, -27.4796) projected
  line L709 (-46.7484, -27.4796) -> (-46.1834, -27.4796) projected
  line L710 (-46.1834, -27.4796) -> (-46.1834, -27.0796) projected
  line L711 (-46.1834, -27.0796) -> (-46.7484, -27.0796) projected
  line L712 (-46.7484, -27.0796) -> (-46.7484, -26.6796) projected
  line L713 (-46.7484, -26.6796) -> (-46.1823, -26.6796) projected
  arc A30 (-45.8834, -25.9746) -> (-46.1823, -26.6796) centre (-45.0834, -26.7296) ccw projected
  line L714 (-45.8834, -25.9746) -> (-45.8834, -25.4046) projected
  line L715 (-45.8834, -25.4046) -> (-44.2834, -25.4046) projected
  line L716 (-44.2834, -25.4046) -> (-44.2834, -25.9746) projected
  arc A31 (-43.9845, -26.6796) -> (-44.2834, -25.9746) centre (-45.0834, -26.7296) ccw projected
  line L717 (-43.9845, -26.6796) -> (-43.4184, -26.6796) projected
  line L718 (-43.4184, -26.6796) -> (-43.4184, -27.0796) projected
  line L719 (-43.4184, -27.0796) -> (-43.9834, -27.0796) projected
  line L720 (-43.9834, -27.0796) -> (-43.9834, -27.4796) projected
  line L721 (-43.9834, -27.4796) -> (-43.4184, -27.4796) projected
  line L722 (-43.4184, -27.4796) -> (-43.4184, -27.8796) projected
  line L723 (-43.4184, -27.8796) -> (-43.9834, -27.8796) projected
  line L724 (-43.9834, -27.8796) -> (-43.9834, -28.2796) projected
  line L725 (-43.9834, -28.2796) -> (-43.4184, -28.2796) projected
  line L726 (-43.4184, -28.2796) -> (-43.4184, -28.6796) projected
  line L727 (-43.4184, -28.6796) -> (-43.9834, -28.6796) projected
  line L728 (-43.9834, -28.6796) -> (-43.9834, -29.0796) projected
  line L729 (-43.9834, -29.0796) -> (-43.4184, -29.0796) projected
  line L730 (-43.4184, -29.0796) -> (-43.4184, -29.4796) projected
  line L731 (-43.4184, -29.4796) -> (-43.9834, -29.4796) projected
  line L732 (-43.9834, -29.4796) -> (-43.9834, -29.8796) projected
  line L733 (-43.9834, -29.8796) -> (-43.4184, -29.8796) projected
  line L734 (-43.4184, -29.8796) -> (-43.4184, -30.2796) projected
  line L735 (-43.4184, -30.2796) -> (-43.9834, -30.2796) projected
  line L736 (-43.9834, -30.2796) -> (-43.9834, -30.6796) projected
  line L737 (-43.9834, -30.6796) -> (-43.4184, -30.6796) projected
  line L738 (-43.4184, -30.6796) -> (-43.4184, -31.0796) projected
  line L739 (-43.4184, -31.0796) -> (-43.9834, -31.0796) projected
  line L740 (-43.9834, -31.0796) -> (-43.9834, -31.4796) projected
  line L741 (-43.9834, -31.4796) -> (-43.4184, -31.4796) projected
  line L742 (-43.4184, -31.4796) -> (-43.4184, -31.8796) projected
  line L743 (-43.4184, -31.8796) -> (-43.9834, -31.8796) projected
  arc A32 (-45.4113, 3.7204) -> (-44.7555, 3.7204) centre (-45.0834, 4.7704) ccw projected
  line L744 (-45.4113, 3.7204) -> (-46.0409, 3.7204) projected
  line L745 (-46.0409, 3.7204) -> (-46.0409, 4.2289) projected
  arc A33 (-46.1834, 4.7704) -> (-46.0409, 4.2289) centre (-45.0834, 4.7704) ccw projected
  line L746 (-46.1834, 4.7704) -> (-46.1834, 4.9954) projected
  line L747 (-46.1834, 4.9954) -> (-46.9059, 4.9954) projected
  line L748 (-46.9059, 4.9954) -> (-46.9059, 5.3954) projected
  line L749 (-46.9059, 5.3954) -> (-46.1834, 5.3954) projected
  line L750 (-46.1834, 5.3954) -> (-46.1834, 5.7954) projected
  line L751 (-46.1834, 5.7954) -> (-46.9059, 5.7954) projected
  line L752 (-46.9059, 5.7954) -> (-46.9059, 6.1954) projected
  line L753 (-46.9059, 6.1954) -> (-46.1834, 6.1954) projected
  line L754 (-46.1834, 6.1954) -> (-46.1834, 6.5954) projected
  line L755 (-46.1834, 6.5954) -> (-46.9059, 6.5954) projected
  line L756 (-46.9059, 6.5954) -> (-46.9059, 6.9954) projected
  line L757 (-46.9059, 6.9954) -> (-46.1834, 6.9954) projected
  line L758 (-46.1834, 6.9954) -> (-46.1834, 7.3954) projected
  line L759 (-46.1834, 7.3954) -> (-46.9059, 7.3954) projected
  line L760 (-46.9059, 7.3954) -> (-46.9059, 7.7954) projected
  line L761 (-46.9059, 7.7954) -> (-46.1834, 7.7954) projected
  line L762 (-46.1834, 7.7954) -> (-46.1834, 8.1954) projected
  line L763 (-46.1834, 8.1954) -> (-46.9059, 8.1954) projected
  line L764 (-46.9059, 8.1954) -> (-46.9059, 8.5954) projected
  line L765 (-46.9059, 8.5954) -> (-46.1834, 8.5954) projected
  line L766 (-46.1834, 8.5954) -> (-46.1834, 8.9954) projected
  line L767 (-46.1834, 8.9954) -> (-46.9059, 8.9954) projected
  line L768 (-46.9059, 8.9954) -> (-46.9059, 9.3954) projected
  line L769 (-46.9059, 9.3954) -> (-46.1834, 9.3954) projected
  line L770 (-46.1834, 9.3954) -> (-46.1834, 9.7954) projected
  line L771 (-46.1834, 9.7954) -> (-46.9059, 9.7954) projected
  line L772 (-46.9059, 9.7954) -> (-46.9059, 10.1954) projected
  line L773 (-46.9059, 10.1954) -> (-46.1834, 10.1954) projected
  line L774 (-46.1834, 10.1954) -> (-46.1834, 10.5954) projected
  line L775 (-46.1834, 10.5954) -> (-46.9059, 10.5954) projected
  line L776 (-46.9059, 10.5954) -> (-46.9059, 10.9954) projected
  line L777 (-46.9059, 10.9954) -> (-46.1343, 10.9954) projected
  arc A34 (-45.6379, 11.6204) -> (-46.1343, 10.9954) centre (-45.0834, 10.6704) ccw projected
  line L778 (-45.6379, 11.6204) -> (-46.0409, 11.6204) projected
  line L779 (-46.0409, 11.6204) -> (-46.0409, 12.2704) projected
  line L780 (-46.0409, 12.2704) -> (-44.4409, 12.2704) projected
  line L781 (-44.4409, 12.2704) -> (-44.4409, 11.6204) projected
  line L782 (-44.4409, 11.6204) -> (-44.5289, 11.6204) projected
  arc A35 (-44.0325, 10.9954) -> (-44.5289, 11.6204) centre (-45.0834, 10.6704) ccw projected
  line L783 (-44.0325, 10.9954) -> (-43.5759, 10.9954) projected
  line L784 (-43.5759, 10.9954) -> (-43.5759, 10.5954) projected
  line L785 (-43.5759, 10.5954) -> (-43.9834, 10.5954) projected
  line L786 (-43.9834, 10.5954) -> (-43.9834, 10.1954) projected
  line L787 (-43.9834, 10.1954) -> (-43.5759, 10.1954) projected
  line L788 (-43.5759, 10.1954) -> (-43.5759, 9.7954) projected
  line L789 (-43.5759, 9.7954) -> (-43.9834, 9.7954) projected
  line L790 (-43.9834, 9.7954) -> (-43.9834, 9.3954) projected
  line L791 (-43.9834, 9.3954) -> (-43.5759, 9.3954) projected
  line L792 (-43.5759, 9.3954) -> (-43.5759, 8.9954) projected
  line L793 (-43.5759, 8.9954) -> (-43.9834, 8.9954) projected
  line L794 (-43.9834, 8.9954) -> (-43.9834, 8.5954) projected
  line L795 (-43.9834, 8.5954) -> (-43.5759, 8.5954) projected
  line L796 (-43.5759, 8.5954) -> (-43.5759, 8.1954) projected
  line L797 (-43.5759, 8.1954) -> (-43.9834, 8.1954) projected
  line L798 (-43.9834, 8.1954) -> (-43.9834, 7.7954) projected
  line L799 (-43.9834, 7.7954) -> (-43.5759, 7.7954) projected
  line L800 (-43.5759, 7.7954) -> (-43.5759, 7.3954) projected
  line L801 (-43.5759, 7.3954) -> (-43.9834, 7.3954) projected
  line L802 (-43.9834, 7.3954) -> (-43.9834, 6.9954) projected
  line L803 (-43.9834, 6.9954) -> (-43.5759, 6.9954) projected
  line L804 (-43.5759, 6.9954) -> (-43.5759, 6.5954) projected
  line L805 (-43.5759, 6.5954) -> (-43.9834, 6.5954) projected
  line L806 (-43.9834, 6.5954) -> (-43.9834, 6.1954) projected
  line L807 (-43.9834, 6.1954) -> (-43.5759, 6.1954) projected
  line L808 (-43.5759, 6.1954) -> (-43.5759, 5.7954) projected
  line L809 (-43.5759, 5.7954) -> (-43.9834, 5.7954) projected
  line L810 (-43.9834, 5.7954) -> (-43.9834, 5.3954) projected
  line L811 (-43.9834, 5.3954) -> (-43.5759, 5.3954) projected
  line L812 (-43.5759, 5.3954) -> (-43.5759, 4.9954) projected
  line L813 (-43.5759, 4.9954) -> (-43.9834, 4.9954) projected
  line L814 (-43.9834, 4.9954) -> (-43.9834, 4.7704) projected
  arc A36 (-44.4409, 3.8775) -> (-43.9834, 4.7704) centre (-45.0834, 4.7704) ccw projected
  line L815 (-44.4409, 3.8775) -> (-44.4409, 3.7204) projected
  line L816 (-44.4409, 3.7204) -> (-44.7555, 3.7204) projected
  arc A37 (-45.4826, 22.4454) -> (-44.6842, 22.4454) centre (-45.0834, 23.4704) ccw projected
  line L817 (-45.4826, 22.4454) -> (-46.1384, 22.4454) projected
  line L818 (-46.1384, 22.4454) -> (-46.1384, 23.0954) projected
  line L819 (-46.1384, 23.0954) -> (-46.1175, 23.0954) projected
  arc A38 (-46.1834, 23.4704) -> (-46.1175, 23.0954) centre (-45.0834, 23.4704) ccw projected
  line L820 (-46.1834, 23.4704) -> (-46.1834, 29.3704) projected
  arc A39 (-45.5927, 30.3454) -> (-46.1834, 29.3704) centre (-45.0834, 29.3704) ccw projected
  line L821 (-45.5927, 30.3454) -> (-46.1384, 30.3454) projected
  line L822 (-46.1384, 30.3454) -> (-46.1384, 30.9954) projected
  line L823 (-46.1384, 30.9954) -> (-44.5384, 30.9954) projected
  line L824 (-44.5384, 30.9954) -> (-44.5384, 30.3454) projected
  line L825 (-44.5384, 30.3454) -> (-44.5741, 30.3454) projected
  arc A40 (-44.0406, 29.7204) -> (-44.5741, 30.3454) centre (-45.0834, 29.3704) ccw projected
  line L826 (-44.0406, 29.7204) -> (-43.6734, 29.7204) projected
  line L827 (-43.6734, 29.7204) -> (-43.6734, 29.3204) projected
  line L828 (-43.6734, 29.3204) -> (-43.9834, 29.3204) projected
  line L829 (-43.9834, 29.3204) -> (-43.9834, 28.9204) projected
  line L830 (-43.9834, 28.9204) -> (-43.6734, 28.9204) projected
  line L831 (-43.6734, 28.9204) -> (-43.6734, 28.5204) projected
  line L832 (-43.6734, 28.5204) -> (-43.9834, 28.5204) projected
  line L833 (-43.9834, 28.5204) -> (-43.9834, 28.1204) projected
  line L834 (-43.9834, 28.1204) -> (-43.6734, 28.1204) projected
  line L835 (-43.6734, 28.1204) -> (-43.6734, 27.7204) projected
  line L836 (-43.6734, 27.7204) -> (-43.9834, 27.7204) projected
  line L837 (-43.9834, 27.7204) -> (-43.9834, 27.3204) projected
  line L838 (-43.9834, 27.3204) -> (-43.6734, 27.3204) projected
  line L839 (-43.6734, 27.3204) -> (-43.6734, 26.9204) projected
  line L840 (-43.6734, 26.9204) -> (-43.9834, 26.9204) projected
  line L841 (-43.9834, 26.9204) -> (-43.9834, 26.5204) projected
  line L842 (-43.9834, 26.5204) -> (-43.6734, 26.5204) projected